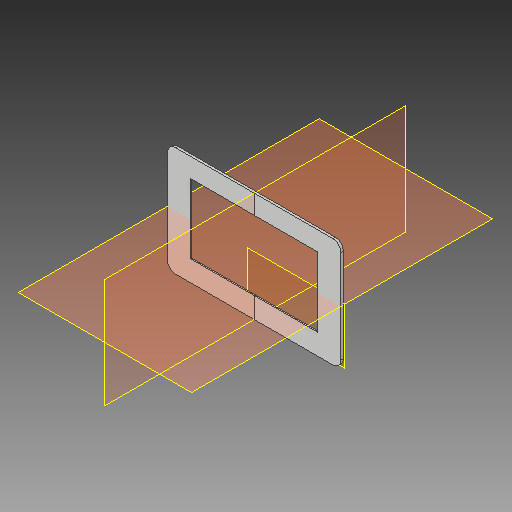
# Autodesk Inventor part: pos cover aug
Saved by Autodesk Inventor 2019.5 (Build 235369000, 369)
## iProperties
Created: 2021-08-27
Part Number: pos cover aug
Material: 일반
Document SubType Name: Modeling
Designer: msj19
Density: 1 g/cm^3
Appearance: 기본값
Author: msj19
Autodesk Inventor part; units mm, degrees
ref_plane "우측면도" through (0, 0, 0) normal (1, 0, 0) x (0, 1, 0)
ref_plane "평면도" through (0, 0, 0) normal (0, 1, 0) x (-1, 0, 0)
ref_plane "정면도" through (0, 0, 0) normal (0, 0, 1) x (1, 0, 0)
ref_plane "작업 평면1" through (12, -15, -1) normal (0, 0, 1) x (1, 0, 0)
sketch "스케치1" plane through (12, -15, -1) normal (0, 0, 1) x (1, 0, 0)
  line L0 (-12, 139.2405) -> (-104.5, 139.2405) projected
  arc A0 (-104.5, 139.2405) -> (-110.5, 133.2405) centre (-104.5, 133.2405) ccw projected
  line L1 (-110.5, 66.2405) -> (-110.5, 16.2405) projected
  arc A1 (-110.5, 16.2405) -> (-104.5, 10.2405) centre (-104.5, 16.2405) ccw projected
  line L2 (-104.5, 10.2405) -> (-12, 10.2405) projected
  line L3 (-110.5, 81.2405) -> (-110.5, 66.2405) projected
  line L4 (-112.5, 133.2405) -> (-112.5, 81.2405) projected
  line L5 (-114.5, 133.2405) -> (-114.5, 81.2405) projected
  arc A2 (-104.5, 143.2405) -> (-114.5, 133.2405) centre (-104.5, 133.2405) ccw projected
  arc A3 (-104.5, 141.2405) -> (-112.5, 133.2405) centre (-104.5, 133.2405) ccw projected
  line L6 (-104.5, 143.2405) -> (-12, 143.2405) projected
  line L7 (-104.5, 139.2405) -> (-12, 139.2405) projected
  line L8 (-12, 141.2405) -> (-104.5, 141.2405) projected
  line L9 (-12, 143.2405) -> (92.5, 143.2405) projected
  line L10 (92.5, 141.2405) -> (-12, 141.2405) projected
  line L11 (100.5, 73.7405) -> (100.5, 133.2405) projected
  arc A4 (100.5, 133.2405) -> (92.5, 141.2405) centre (92.5, 133.2405) ccw projected
  line L12 (92.5, 141.2405) -> (-12, 141.2405) projected
  line L13 (-12, 139.2405) -> (92.5, 139.2405) projected
  arc A5 (98.5, 133.2405) -> (92.5, 139.2405) centre (92.5, 133.2405) ccw projected
  line L14 (98.5, 133.2405) -> (98.5, 73.7405) projected
  line L15 (102.5, 73.7405) -> (102.5, 133.2405) projected
  arc A6 (102.5, 133.2405) -> (92.5, 143.2405) centre (92.5, 133.2405) ccw projected
  line L16 (-12, 143.2405) -> (92.5, 143.2405) projected
  line L17 (-12, 141.2405) -> (92.5, 141.2405) projected
  arc A7 (100.5, 133.2405) -> (92.5, 141.2405) centre (92.5, 133.2405) ccw projected
  line L18 (100.5, 133.2405) -> (100.5, 73.7405) projected
  line L19 (98.5, 73.7405) -> (98.5, 16.2405) projected
  arc A8 (92.5, 10.2405) -> (98.5, 16.2405) centre (92.5, 16.2405) ccw projected
  line L20 (92.5, 10.2405) -> (-12, 10.2405) projected
  line L21 (-12, 8.2405) -> (92.5, 8.2405) projected
  arc A9 (92.5, 8.2405) -> (100.5, 16.2405) centre (92.5, 16.2405) ccw projected
  line L22 (100.5, 16.2405) -> (100.5, 73.7405) projected
  arc A10 (92.5, 6.2405) -> (102.5, 16.2405) centre (92.5, 16.2405) ccw projected
  line L23 (102.5, 16.2405) -> (102.5, 73.7405) projected
  line L24 (100.5, 73.7405) -> (100.5, 16.2405) projected
  arc A11 (92.5, 8.2405) -> (100.5, 16.2405) centre (92.5, 16.2405) ccw projected
  line L25 (92.5, 8.2405) -> (-12, 8.2405) projected
  line L26 (92.5, 6.2405) -> (-12, 6.2405) projected
  arc A12 (-114.5, 16.2405) -> (-104.5, 6.2405) centre (-104.5, 16.2405) ccw projected
  line L27 (-104.5, 6.2405) -> (-12, 6.2405) projected
  line L28 (-12, 8.2405) -> (-104.5, 8.2405) projected
  arc A13 (-112.5, 16.2405) -> (-104.5, 8.2405) centre (-104.5, 16.2405) ccw projected
  line L29 (-112.5, 16.2405) -> (-112.5, 66.2405) projected
  line L30 (-114.5, 66.2405) -> (-114.5, 16.2405) projected
  line L31 (-112.5, 66.2405) -> (-112.5, 16.2405) projected
  arc A14 (-112.5, 16.2405) -> (-104.5, 8.2405) centre (-104.5, 16.2405) ccw projected
  line L32 (-104.5, 8.2405) -> (-12, 8.2405) projected
  line L33 (-12, 10.2405) -> (-104.5, 10.2405) projected
  arc A15 (-110.5, 16.2405) -> (-104.5, 10.2405) centre (-104.5, 16.2405) ccw projected
  line L34 (-110.5, 16.2405) -> (-110.5, 66.2405) projected
  line L35 (-112.5, 66.2405) -> (-112.5, 16.2405) projected
  arc A16 (-112.5, 16.2405) -> (-104.5, 8.2405) centre (-104.5, 16.2405) ccw projected
  line L36 (-104.5, 8.2405) -> (-12, 8.2405) projected
  line L37 (-12, 10.2405) -> (-104.5, 10.2405) projected
  arc A17 (-110.5, 16.2405) -> (-104.5, 10.2405) centre (-104.5, 16.2405) ccw projected
  line L38 (-110.5, 16.2405) -> (-110.5, 66.2405) projected
  arc A18 (-114.5, 16.2405) -> (-104.5, 6.2405) centre (-104.5, 16.2405) ccw projected
  line L39 (-104.5, 6.2405) -> (-12, 6.2405) projected
  line L40 (-12, 8.2405) -> (-104.5, 8.2405) projected
  arc A19 (-112.5, 16.2405) -> (-104.5, 8.2405) centre (-104.5, 16.2405) ccw projected
  line L41 (-112.5, 16.2405) -> (-112.5, 66.2405) projected
  line L42 (-114.5, 66.2405) -> (-114.5, 16.2405) projected
  line L43 (-112.5, 66.2405) -> (-112.5, 16.2405) projected
  line L44 (-12, 10.2405) -> (-104.5, 10.2405) projected
  line L45 (-114.5, 81.2405) -> (-114.5, 66.2405) projected
  line L46 (-112.5, 81.2405) -> (-112.5, 66.2405) projected
  line L47 (-112.5, 81.2405) -> (-112.5, 66.2405) projected
  line L48 (-110.5, 81.2405) -> (-110.5, 66.2405) projected
  line L49 (-112.5, 81.2405) -> (-112.5, 66.2405) projected
  line L50 (-112.5, 66.2405) -> (-112.5, 16.2405) projected
  line L51 (-110.5, 81.2405) -> (-110.5, 133.2405) projected
  line L52 (-85.5, 119.2405) -> (73.5, 119.2405)
  line L53 (73.5, 119.2405) -> (73.5, 32.2405)
  line L54 (73.5, 32.2405) -> (-85.5, 32.2405)
  line L55 (-85.5, 32.2405) -> (-85.5, 119.2405)
  dimension "d0" = 20
  dimension "d1" = 25
  dimension "d3" = 25
  dimension "d4" = 22
  constraints: 8 end point, 2 parallel, 1 horizontal, 1 perpendicular
  measures "d0" distance between parallel lines of L52 L0
  measures "d1" distance between parallel lines of L51 L55
  measures "d3" distance between parallel lines of L14 L53
  measures "d4" distance between parallel lines of L20 L54
extrude "돌출1" add sketch "스케치1" along normal blind 3 contours L13 A5 L14 L19 A8 L20 L2 A1 L1 L3 L51 A0 L0 | A3 L8 L10 A4 L11 L22 A9 L21 L28 A13 L29 L46 L4 | A2 L6 L9 A6 L15 L23 A10 L26 L27 A12 L30 L45 L5
sketch "스케치2" plane through (12, -15, -1) normal (0, 0, -1) x (-1, 0, 0)
  line L0 (-92.5, 141.2405) -> (12, 141.2405) projected
  line L1 (12, 139.2405) -> (-92.5, 139.2405) projected
  arc A0 (-92.5, 141.2405) -> (-100.5, 133.2405) centre (-92.5, 133.2405) ccw projected
  arc A1 (-92.5, 139.2405) -> (-98.5, 133.2405) centre (-92.5, 133.2405) ccw projected
  line L2 (-98.5, 133.2405) -> (-98.5, 73.7405) projected
  line L3 (-100.5, 73.7405) -> (-100.5, 133.2405) projected
  arc A2 (-100.5, 16.2405) -> (-92.5, 8.2405) centre (-92.5, 16.2405) ccw projected
  arc A3 (-98.5, 16.2405) -> (-92.5, 10.2405) centre (-92.5, 16.2405) ccw projected
  line L4 (-92.5, 10.2405) -> (12, 10.2405) projected
  line L5 (12, 8.2405) -> (-92.5, 8.2405) projected
  line L6 (104.5, 10.2405) -> (12, 10.2405) projected
  line L7 (12, 8.2405) -> (104.5, 8.2405) projected
  arc A4 (104.5, 8.2405) -> (112.5, 16.2405) centre (104.5, 16.2405) ccw projected
  arc A5 (104.5, 10.2405) -> (110.5, 16.2405) centre (104.5, 16.2405) ccw projected
  line L8 (110.5, 66.2405) -> (110.5, 16.2405) projected
  line L9 (112.5, 16.2405) -> (112.5, 66.2405) projected
  line L10 (110.5, 81.2405) -> (110.5, 133.2405) projected
  line L11 (112.5, 133.2405) -> (112.5, 81.2405) projected
  arc A6 (112.5, 133.2405) -> (104.5, 141.2405) centre (104.5, 133.2405) ccw projected
  arc A7 (110.5, 133.2405) -> (104.5, 139.2405) centre (104.5, 133.2405) ccw projected
  line L12 (12, 139.2405) -> (104.5, 139.2405) projected
  line L13 (12, 141.2405) -> (104.5, 141.2405) projected
  line L14 (-100.5, 73.7405) -> (-100.5, 16.2405)
  line L15 (-98.5, 73.7405) -> (-98.5, 16.2405)
  line L16 (110.5, 81.2405) -> (110.5, 66.2405)
  line L17 (112.5, 81.2405) -> (112.5, 66.2405)
  point P0 (12, 15)
  constraints: 8 end point, 2 parallel, 2 vertical
extrude "돌출2" cut sketch "스케치2" against normal blind 1.5
sketch "스케치3" plane through (12, -15, -1) normal (0, 0, -1) x (-1, 0, 0)
  line L0 (-73.5, 119.2405) -> (85.5, 119.2405) projected
  line L1 (-73.5, 32.2405) -> (-73.5, 119.2405) projected
  line L2 (85.5, 32.2405) -> (-73.5, 32.2405) projected
  line L3 (85.5, 119.2405) -> (85.5, 32.2405) projected
  line L4 (105.5, 131.2405) -> (-93.5, 131.2405)
  line L5 (-93.5, 131.2405) -> (-93.5, 18.2405)
  line L6 (-93.5, 18.2405) -> (105.5, 18.2405)
  line L7 (105.5, 18.2405) -> (105.5, 131.2405)
  line L8 (-92.5, 143.2405) -> (104.5, 143.2405) projected
  line L9 (104.5, 6.2405) -> (-92.5, 6.2405) projected
  line L10 (-102.5, 16.2405) -> (-102.5, 133.2405) projected
  line L11 (114.5, 133.2405) -> (114.5, 16.2405) projected
  arc A0 (-92.5, 139.2405) -> (-98.5, 133.2405) centre (-92.5, 133.2405) ccw projected
  line L12 (-98.5, 133.2405) -> (-98.5, 16.2405) projected
  arc A1 (-98.5, 16.2405) -> (-92.5, 10.2405) centre (-92.5, 16.2405) ccw projected
  line L13 (-92.5, 10.2405) -> (104.5, 10.2405) projected
  arc A2 (104.5, 10.2405) -> (110.5, 16.2405) centre (104.5, 16.2405) ccw projected
  line L14 (110.5, 16.2405) -> (110.5, 133.2405) projected
  arc A3 (110.5, 133.2405) -> (104.5, 139.2405) centre (104.5, 133.2405) ccw projected
  line L15 (104.5, 139.2405) -> (-92.5, 139.2405) projected
  line L16 (-73.5, 32.2405) -> (-73.5, 119.2405) projected
  line L17 (-73.5, 119.2405) -> (85.5, 119.2405) projected
  line L18 (85.5, 119.2405) -> (85.5, 32.2405) projected
  line L19 (85.5, 32.2405) -> (-73.5, 32.2405) projected
  point P0 (12, 15)
  dimension "d14" = 5
  dimension "d15" = 8
  dimension "d16" = 5
  dimension "d17" = 8
  constraints: 8 end point
  measures "d14" distance between parallel lines of L12 L5
  measures "d15" distance between parallel lines of L15 L4
  measures "d16" distance between parallel lines of L14 L7
  measures "d17" distance between parallel lines of L13 L6
extrude "돌출3" cut sketch "스케치3" against normal blind 1.5 contours L7 L6 L5 L4
sketch "스케치4" plane through (12, -15, 0.5) normal (0, 0, -1) x (-1, 0, 0)
  line L0 (-92.5, 143.2405) -> (104.5, 143.2405) projected
  line L1 (104.5, 6.2405) -> (-92.5, 6.2405) projected
  line L2 (-102.5, 16.2405) -> (-102.5, 133.2405) projected
  line L3 (114.5, 133.2405) -> (114.5, 16.2405) projected
  line L4 (6, 143.2405) -> (6, 6.2405)
  line L5 (-102.5, 74.7405) -> (114.5, 74.7405)
  point P0 (12, 15)
  constraints: 4 end point, 4 midpoint
surface extrude "돌출 곡면1" sketch "스케치4" along normal mid plane 376.75 shown yes curves L4
sketch "스케치5" plane through (12, -15, 0.5) normal (0, 0, -1) x (-1, 0, 0)
  line L0 (-102.5, 16.2405) -> (-102.5, 133.2405) projected
  line L1 (114.5, 133.2405) -> (114.5, 16.2405) projected
  line L2 (-102.5, 74.7405) -> (114.5, 74.7405)
  point P0 (12, 15)
  constraints: 2 end point, 2 midpoint
surface extrude "돌출 곡면2" sketch "스케치5" along normal mid plane 376.75 shown yes curves L2
split body "분할1" result two bodies by surface "돌출 곡면1" first body at (-92.8333, 45.5738, 1.5)
body "Srf1"
body "Srf2"
